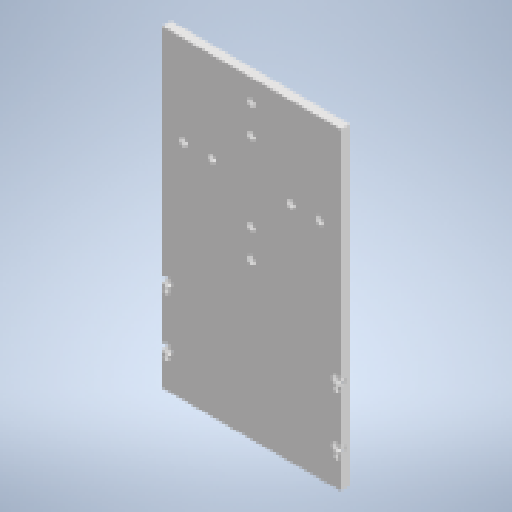
# Autodesk Inventor part: 290x200(10li)
Saved by Autodesk Inventor 2023 (Build 270158000, 158)
## iProperties
Created: 2025-04-11
Part Number: 290x200(10li)
Material: Generic
Document SubType Name: Modeling
Designer: huyqu
Density: 1 g/cm^3
Appearance: Default
Author: huyqu
Autodesk Inventor part; units mm, degrees
ref_plane "YZ Plane" through (0, 0, 0) normal (1, 0, 0) x (0, 1, 0)
ref_plane "XZ Plane" through (0, 0, 0) normal (0, 1, 0) x (-1, 0, 0)
ref_plane "XY Plane" through (0, 0, 0) normal (0, 0, 1) x (1, 0, 0)
sketch "Sketch1" plane through (0, 0, 0) normal (0, 0, 1) x (1, 0, 0)
  line L0 (0, 0) -> (200, 0)
  line L1 (200, 0) -> (200, 350)
  line L2 (200, 350) -> (0, 350)
  line L3 (0, 350) -> (0, 0)
  dimension "d0" = 200
  dimension "d1" = 350
  constraints: 8 end point, 2 parallel, 1 horizontal, 1 perpendicular
  measures "d0" distance of L0.start L0.end
  measures "d1" distance of L0.end L1.end
extrude "Extrusion1" add sketch "Sketch1" along normal blind 10
sketch "Sketch2" plane through (0, 0, 10) normal (0, 0, 1) x (1, 0, 0)
  circle A0 centre (144, 250) radius 2.067 projected
  circle A1 centre (176, 250) radius 2.067 projected
  circle A2 centre (100, 326) radius 2.067 projected
  circle A3 centre (100, 294) radius 2.067 projected
  circle A4 centre (56, 250) radius 2.067 projected
  circle A5 centre (24, 250) radius 2.067 projected
  circle A6 centre (100, 206) radius 2.067 projected
  circle A7 centre (100, 174) radius 2.067 projected
  point P0 (0, 0)
hole "Hole1" at (24, 250, 10) at (56, 250, 10) at (100, 294, 10) at (100, 326, 10) at (144, 250, 10) at (176, 250, 10) at (100, 206, 10) at (100, 174, 10) direction (0, 0, -1) diameter 6 end through all counterbore diameter 9 counterbore depth 5
sketch "Sketch3" plane through (0, 0, 0) normal (0, -1, 0) x (1, 0, 0)
  line L0 (0, 0) -> (0, 10) projected
  line L1 (0, 5) -> (200, 5)
  line L2 (200, 0) -> (200, 10) projected
  circle A0 centre (24, 5) radius 3
  circle A1 centre (56, 5) radius 3
  circle A2 centre (144, 5) radius 3
  circle A3 centre (176, 5) radius 3
  dimension "d11" = 6
  dimension "d12" = 6
  dimension "d13" = 6
  dimension "d14" = 6
  dimension "d15" = 24
  dimension "d16" = 56
  dimension "d17" = 24
  dimension "d18" = 56
  constraints: 4 centre point, 2 end point, 2 midpoint, 1 point on line
  measures "d11" diameter of A0
  measures "d12" diameter of A1
  measures "d13" diameter of A2
  measures "d14" diameter of A3
  measures "d15" distance from line of A0.centre L0
  measures "d16" distance from line of A1.centre L0
  measures "d17" distance from line of L2 A3.centre
  measures "d18" distance from line of L2 A2.centre
hole "Hole2" at (24, 0, 5) at (56, 0, 5) at (144, 0, 5) at (176, 0, 5) direction (0, 1, 0) diameter 4.917 depth 17.1 thread size "M6x1" class "6H" standard "ISO Metric profile"
sketch "Sketch4" plane through (0, 0, 10) normal (0, 0, 1) x (1, 0, 0)
  circle A0 centre (195, 40) radius 2.5941 projected
  circle A1 centre (195, 105) radius 2.5941 projected
  circle A2 centre (5, 105) radius 2.5941 projected
  circle A3 centre (5, 40) radius 2.5941 projected
  point P0 (0, 0)
hole "Hole3" at (5, 105, 10) at (5, 40, 10) at (195, 105, 10) at (195, 40, 10) direction (0, 0, -1) diameter 7 end through all counterbore diameter 11 counterbore depth 5
sketch "Sketch7" plane through (0, 0, 0) normal (0, 0, -1) x (-1, 0, 0)
  circle A0 centre (-195, 93) radius 2.4585
  circle A1 centre (-195, 28) radius 2.4585
  circle A2 centre (-5, 92.9758) radius 2.4585
  circle A3 centre (-5, 27.9758) radius 2.4585
  point P0 (0, 0)
  constraints: 4 centre point, 8 other
hole "Hole6" at (195, 93, 0) at (5, 92.9758, 0) at (5, 27.9758, 0) at (195, 28, 0) direction (0, 0, 1) diameter 6 end through all counterbore diameter 10 counterbore depth 5
body "Solid1"
